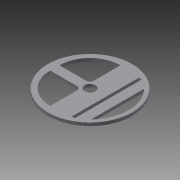
# Autodesk Inventor part: fixpart
Saved by Autodesk Inventor 2015 (Build 190159000, 159)
## iProperties
Created: 2015-02-18
Part Number: fixpart
Material: Generic
Document SubType Name: Modeling
Designer: Hanjie
Density: 1 g/cm^3
Appearance: Default
Author: Hanjie
Autodesk Inventor part; units mm, degrees
ref_plane "YZ Plane" through (0, 0, 0) normal (1, 0, 0) x (0, 1, 0)
ref_plane "XZ Plane" through (0, 0, 0) normal (0, 1, 0) x (-1, 0, 0)
ref_plane "XY Plane" through (0, 0, 0) normal (0, 0, 1) x (1, 0, 0)
sketch "Sketch1" plane through (0, 0, 0) normal (0, 1, 0) x (-1, 0, 0)
  circle A0 centre (0, 0) radius 34.925
  dimension "d0" = 69.85
  constraints: 1 centre point, 1 coincident
  measures "d0" diameter of A0
extrude "Extrusion1" add sketch "Sketch1" along normal blind 2.54
sketch "Sketch2" plane through (0, 0, 0) normal (0, -1, 0) x (1, 0, 0)
  line L0 (0, 0) -> (15.24, 0)
  line L1 (15.24, 0) -> (15.24, -27.94)
  line L2 (15.24, -27.94) -> (12.7, -27.94)
  line L3 (12.7, -27.94) -> (12.7, 27.94)
  line L4 (12.7, 27.94) -> (15.24, 27.94)
  line L5 (15.24, 27.94) -> (15.24, -27.94)
  line L6 (0, 0) -> (0, -3.81)
  line L7 (0, -3.81) -> (-3.81, -3.81)
  arc A0 (-3.81, -6.985) -> (-6.985, -3.81) centre (-6.985, -6.985) ccw
  arc A1 (-29.21, -3.81) -> (-3.81, -29.21) centre (-3.81, -3.81) ccw
  line L8 (-3.81, -3.81) -> (-3.81, -29.21) construction
  line L9 (-3.81, -3.81) -> (-29.21, -3.81) construction
  line L10 (-3.81, -29.21) -> (-3.81, -6.985)
  line L11 (-29.21, -3.81) -> (-6.985, -3.81)
  circle A2 centre (0, 0) radius 34.925 projected
  line L12 (-34.925, 0) -> (0, 0)
  arc A3 (-6.985, 3.81) -> (-3.81, 6.985) centre (-6.985, 6.985) ccw
  arc A4 (-3.81, 29.21) -> (-29.21, 3.81) centre (-3.81, 3.81) ccw
  line L13 (-3.81, 3.81) -> (-3.81, 29.21) construction
  line L14 (-3.81, 3.81) -> (-29.21, 3.81) construction
  line L15 (-6.985, 3.81) -> (-29.21, 3.81)
  line L16 (-3.81, 6.985) -> (-3.81, 29.21)
  line L17 (15.24, 0) -> (22.86, 0)
  line L18 (22.86, 0) -> (22.86, -22.0337)
  line L19 (22.86, 22.0337) -> (22.86, 0)
  arc A5 (15.0804, -27.94) -> (15.24, -27.8533) centre (0, 0) ccw
  arc A6 (22.86, -22.0337) -> (22.86, 22.0337) centre (0, 0) ccw
  arc A7 (15.24, 27.8533) -> (15.0804, 27.94) centre (0, 0) ccw
  circle A8 centre (0, 0) radius 4.445
  dimension "d3" = 15.24
  dimension "d4" = 27.94
  dimension "d5" = 2.54
  dimension "d6" = 55.88
  dimension "d7" = 3.81
  dimension "d8" = 3.81
  dimension "d9" = 25.4
  dimension "d11" = 3.175
  dimension "d13" = 25.4
  dimension "d14" = 90
  dimension "d19" = 7.62
  dimension "d20" = 8.89
  constraints: 40 end point, 14 point on circle, 8 centre point, 8 symmetric about line, 6 point on line, 4 horizontal, 3 coincident, 3 parallel, 3 perpendicular, 3 vertical, 2 collinear, 1 horizontal alignment, 3 other
  measures "d3" distance of L0.start L0.end
  measures "d4" distance of L0.end L1.end
  measures "d5" distance of L3.end L4.end
  measures "d6" distance of L2.end L3.end
  measures "d7" distance of L0.start L6.end
  measures "d8" distance of L6.end L7.end
  measures "d9" distance of L7.end L9.end
  measures "d11" radius of A0
  measures "d13" radius of A1
  measures "d14" angle of L9 L8
  measures "d19" distance of L0.end L17.end
  measures "d20" diameter of A8
extrude "Extrusion2" cut sketch "Sketch2" against normal blind 2.54 contours L12 A8 L0 | L0 A8 L7 L6 | L6 L7 A8 L12 | L19 A6 L18 | L3 L4 A7 L5 L0 | L0 L1 A5 L2 L3 | L1 L2 A5 | A7 L4 L5 | L10 A1 L11 A0 | L15 A4 L16 A3
body "Solid1"
